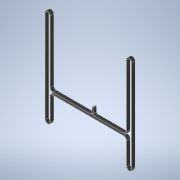
# Autodesk Inventor part: GT2 Belt
Saved by Autodesk Inventor 2022 (Build 260153000, 153)
## iProperties
Created: 2022-06-12
Part Number: GT2 Belt
Material: Generic
Document SubType Name: Modeling
Designer: Nick
Density: 1 g/cm^3
Appearance: Default
Author: Nick
Autodesk Inventor part; units mm, degrees
ref_plane "YZ Plane" through (0, 0, 0) normal (1, 0, 0) x (0, 1, 0)
ref_plane "XZ Plane" through (0, 0, 0) normal (0, 1, 0) x (-1, 0, 0)
ref_plane "XY Plane" through (0, 0, 0) normal (0, 0, 1) x (1, 0, 0)
ref_plane "Work Plane1" through (-134.646947, -237.429887, -822.943102) normal (0, 0, -1) x (0, -1, 0)
ref_plane "Work Plane3" through (-197.934852, -177.205039, -822.943102) normal (0, 1, 0) x (-1, 0, 0)
sketch "Sketch3" plane through (-197.934852, -177.205039, -822.943102) normal (0, 1, 0) x (-1, 0, 0)
  line L0 (0, 0) -> (1, 0)
  line L1 (1, 0) -> (1, -6)
  line L2 (1, -6) -> (0, -6)
  line L3 (0, -6) -> (0, 0)
  point P0 (-197.934852, 822.943102)
  dimension "d10" = 1
  dimension "d11" = 6
  constraints: 8 end point, 2 parallel, 1 horizontal, 1 perpendicular
  measures "d10" distance of L1.end L2.end
  measures "d11" distance of L0.end L1.end
sketch "Sketch1" plane through (-134.646947, -237.429887, -822.943102) normal (0, 0, -1) x (0, -1, 0)
  line L0 (0, 4.84) -> (-39.224848, 4.84)
  line L1 (-43.884848, 9.5) -> (-43.884848, 134.5)
  line L2 (-48.564848, 134.5) -> (-48.564848, 67.627904)
  line L3 (-48.564848, 61.127904) -> (-48.564848, 9.5)
  line L4 (-163, 4.84) -> (-53.224848, 4.84)
  line L5 (-163, -4.84) -> (0, -4.84)
  circle A0 centre (-53.224848, 9.5) radius 4.5 construction
  circle A1 centre (-39.224848, 9.5) radius 4.5 construction
  circle A2 centre (-53.224848, 134.5) radius 4.5
  circle A3 centre (-39.224848, 134.5) radius 4.5
  circle A4 centre (-163, 0) radius 4.5 construction
  circle A5 centre (-163, 144) radius 4.5
  arc A6 (1.927206, 148.234735) -> (2.866938, 147.664391) centre (2.386662, 147.93241) ccw construction
  arc A7 (3.109447, 147.709035) -> (2.866938, 147.664391) centre (3.006655, 147.586422) ccw construction
  arc A8 (3.424444, 147.420348) -> (3.109447, 147.709035) centre (0, 144) ccw construction
  arc A9 (3.401069, 147.174875) -> (3.424444, 147.420348) centre (3.31124, 147.307279) ccw construction
  arc A10 (3.401069, 147.174875) -> (4.051008, 146.288326) centre (3.709856, 146.719737) ccw construction
  arc A11 (4.292141, 146.236767) -> (4.051008, 146.288326) centre (4.150252, 146.162825) ccw construction
  arc A12 (4.472685, 145.849511) -> (4.292141, 146.236767) centre (0, 144) ccw construction
  arc A13 (4.35715, 145.631669) -> (4.472685, 145.849511) centre (4.324827, 145.788371) ccw construction
  arc A14 (4.35715, 145.631669) -> (4.618347, 144.563884) centre (4.468258, 145.093009) ccw construction
  arc A15 (4.821395, 144.423973) -> (4.618347, 144.563884) centre (4.66201, 144.409957) ccw construction
  arc A16 (4.839999, 143.997103) -> (4.821395, 144.423973) centre (0, 144) ccw construction
  arc A17 (4.649894, 143.840057) -> (4.839999, 143.997103) centre (4.679999, 143.997199) ccw construction
  arc A18 (4.649894, 143.840057) -> (4.482586, 142.753596) centre (4.546409, 143.29988) ccw construction
  arc A19 (4.616635, 142.546632) -> (4.482586, 142.753596) centre (4.464019, 142.594677) ccw construction
  arc A20 (4.470468, 142.145136) -> (4.616635, 142.546632) centre (0, 144) ccw construction
  arc A21 (4.234735, 142.072794) -> (4.470468, 142.145136) centre (4.322684, 142.206454) ccw construction
  arc A22 (4.234735, 142.072794) -> (3.664391, 141.133062) centre (3.93241, 141.613338) ccw construction
  arc A23 (3.709035, 140.890553) -> (3.664391, 141.133062) centre (3.586422, 140.993345) ccw construction
  arc A24 (3.420348, 140.575556) -> (3.709035, 140.890553) centre (0, 144) ccw construction
  arc A25 (3.174875, 140.598931) -> (3.420348, 140.575556) centre (3.307279, 140.68876) ccw construction
  arc A26 (3.174875, 140.598931) -> (2.288326, 139.948992) centre (2.719737, 140.290144) ccw construction
  arc A27 (2.236767, 139.707859) -> (2.288326, 139.948992) centre (2.162825, 139.849748) ccw construction
  arc A28 (1.849511, 139.527315) -> (2.236767, 139.707859) centre (0, 144) ccw construction
  arc A29 (1.631669, 139.64285) -> (1.849511, 139.527315) centre (1.788371, 139.675173) ccw construction
  arc A30 (1.631669, 139.64285) -> (0.563884, 139.381653) centre (1.093009, 139.531742) ccw construction
  arc A31 (0.423973, 139.178605) -> (0.563884, 139.381653) centre (0.409957, 139.33799) ccw construction
  arc A32 (-0.002897, 139.160001) -> (0.423973, 139.178605) centre (0, 144) ccw construction
  arc A33 (-0.159943, 139.350106) -> (-0.002897, 139.160001) centre (-0.002801, 139.320001) ccw construction
  arc A34 (-0.159943, 139.350106) -> (-1.246404, 139.517414) centre (-0.70012, 139.453591) ccw construction
  arc A35 (-1.453368, 139.383365) -> (-1.246404, 139.517414) centre (-1.405323, 139.535981) ccw construction
  arc A36 (-1.854864, 139.529532) -> (-1.453368, 139.383365) centre (0, 144) ccw construction
  arc A37 (-1.927206, 139.765265) -> (-1.854864, 139.529532) centre (-1.793546, 139.677316) ccw construction
  arc A38 (-1.927206, 139.765265) -> (-2.866938, 140.335609) centre (-2.386662, 140.06759) ccw construction
  arc A39 (-3.109447, 140.290965) -> (-2.866938, 140.335609) centre (-3.006655, 140.413578) ccw construction
  arc A40 (-3.424444, 140.579652) -> (-3.109447, 140.290965) centre (0, 144) ccw construction
  arc A41 (-3.401069, 140.825125) -> (-3.424444, 140.579652) centre (-3.31124, 140.692721) ccw construction
  arc A42 (-3.401069, 140.825125) -> (-4.051008, 141.711674) centre (-3.709856, 141.280263) ccw construction
  arc A43 (-4.292141, 141.763233) -> (-4.051008, 141.711674) centre (-4.150252, 141.837175) ccw construction
  arc A44 (-4.472685, 142.150489) -> (-4.292141, 141.763233) centre (0, 144) ccw construction
  arc A45 (-4.35715, 142.368331) -> (-4.472685, 142.150489) centre (-4.324827, 142.211629) ccw construction
  arc A46 (-4.35715, 142.368331) -> (-4.618347, 143.436116) centre (-4.468258, 142.906991) ccw construction
  arc A47 (-4.821395, 143.576027) -> (-4.618347, 143.436116) centre (-4.66201, 143.590043) ccw construction
  arc A48 (-4.839999, 144.002897) -> (-4.821395, 143.576027) centre (0, 144) ccw construction
  arc A49 (-4.649894, 144.159943) -> (-4.839999, 144.002897) centre (-4.679999, 144.002801) ccw construction
  arc A50 (-4.649894, 144.159943) -> (-4.482586, 145.246404) centre (-4.546409, 144.70012) ccw construction
  arc A51 (-4.616635, 145.453368) -> (-4.482586, 145.246404) centre (-4.464019, 145.405323) ccw construction
  arc A52 (-4.470468, 145.854864) -> (-4.616635, 145.453368) centre (0, 144) ccw construction
  arc A53 (-4.234735, 145.927206) -> (-4.470468, 145.854864) centre (-4.322684, 145.793546) ccw construction
  arc A54 (-4.234735, 145.927206) -> (-3.664391, 146.866938) centre (-3.93241, 146.386662) ccw construction
  arc A55 (-3.709035, 147.109447) -> (-3.664391, 146.866938) centre (-3.586422, 147.006655) ccw construction
  arc A56 (-3.420348, 147.424444) -> (-3.709035, 147.109447) centre (0, 144) ccw construction
  arc A57 (-3.174875, 147.401069) -> (-3.420348, 147.424444) centre (-3.307279, 147.31124) ccw construction
  arc A58 (-3.174875, 147.401069) -> (-2.288326, 148.051008) centre (-2.719737, 147.709856) ccw construction
  arc A59 (-2.236767, 148.292141) -> (-2.288326, 148.051008) centre (-2.162825, 148.150252) ccw construction
  arc A60 (-1.849511, 148.472685) -> (-2.236767, 148.292141) centre (0, 144) ccw construction
  arc A61 (-1.631669, 148.35715) -> (-1.849511, 148.472685) centre (-1.788371, 148.324827) ccw construction
  arc A62 (-1.631669, 148.35715) -> (-0.563884, 148.618347) centre (-1.093009, 148.468258) ccw construction
  arc A63 (-0.423973, 148.821395) -> (-0.563884, 148.618347) centre (-0.409957, 148.66201) ccw construction
  arc A64 (0.002897, 148.839999) -> (-0.423973, 148.821395) centre (0, 144) ccw construction
  arc A65 (0.159943, 148.649894) -> (0.002897, 148.839999) centre (0.002801, 148.679999) ccw construction
  arc A66 (0.159943, 148.649894) -> (1.246404, 148.482586) centre (0.70012, 148.546409) ccw construction
  arc A67 (1.453368, 148.616635) -> (1.246404, 148.482586) centre (1.405323, 148.464019) ccw construction
  arc A68 (1.854864, 148.470468) -> (1.453368, 148.616635) centre (0, 144) ccw construction
  arc A69 (1.927206, 148.234735) -> (1.854864, 148.470468) centre (1.793546, 148.322684) ccw construction
  arc A70 (3.655529, -2.878229) -> (2.878229, -3.655529) centre (3.252691, -3.252691) ccw construction
  arc A71 (2.863972, -3.9017) -> (2.878229, -3.655529) centre (2.769295, -3.772718) ccw construction
  arc A72 (2.508706, -4.139081) -> (2.863972, -3.9017) centre (0, 0) ccw construction
  arc A73 (2.275818, -4.058048) -> (2.508706, -4.139081) centre (2.425774, -4.002252) ccw construction
  arc A74 (2.275818, -4.058048) -> (1.260227, -4.478719) centre (1.760344, -4.249846) ccw construction
  arc A75 (1.152849, -4.700696) -> (1.260227, -4.478719) centre (1.114738, -4.545301) ccw construction
  arc A76 (0.733785, -4.784053) -> (1.152849, -4.700696) centre (0, 0) ccw construction
  arc A77 (0.549634, -4.620065) -> (0.733785, -4.784053) centre (0.709527, -4.625902) ccw construction
  arc A78 (0.549634, -4.620065) -> (-0.549634, -4.620065) centre (0, -4.6) ccw construction
  arc A79 (-0.733785, -4.784053) -> (-0.549634, -4.620065) centre (-0.709527, -4.625902) ccw construction
  arc A80 (-1.152849, -4.700696) -> (-0.733785, -4.784053) centre (0, 0) ccw construction
  arc A81 (-1.260227, -4.478719) -> (-1.152849, -4.700696) centre (-1.114738, -4.545301) ccw construction
  arc A82 (-1.260227, -4.478719) -> (-2.275818, -4.058048) centre (-1.760344, -4.249846) ccw construction
  arc A83 (-2.508706, -4.139081) -> (-2.275818, -4.058048) centre (-2.425774, -4.002252) ccw construction
  arc A84 (-2.863972, -3.9017) -> (-2.508706, -4.139081) centre (0, 0) ccw construction
  arc A85 (-2.878229, -3.655529) -> (-2.863972, -3.9017) centre (-2.769295, -3.772718) ccw construction
  arc A86 (-2.878229, -3.655529) -> (-3.655529, -2.878229) centre (-3.252691, -3.252691) ccw construction
  arc A87 (-3.9017, -2.863972) -> (-3.655529, -2.878229) centre (-3.772718, -2.769295) ccw construction
  arc A88 (-4.139081, -2.508706) -> (-3.9017, -2.863972) centre (0, 0) ccw construction
  arc A89 (-4.058048, -2.275818) -> (-4.139081, -2.508706) centre (-4.002252, -2.425774) ccw construction
  arc A90 (-4.058048, -2.275818) -> (-4.478719, -1.260227) centre (-4.249846, -1.760344) ccw construction
  arc A91 (-4.700696, -1.152849) -> (-4.478719, -1.260227) centre (-4.545301, -1.114738) ccw construction
  arc A92 (-4.784053, -0.733785) -> (-4.700696, -1.152849) centre (0, 0) ccw construction
  arc A93 (-4.620065, -0.549634) -> (-4.784053, -0.733785) centre (-4.625902, -0.709527) ccw construction
  arc A94 (-4.620065, -0.549634) -> (-4.620065, 0.549634) centre (-4.6, 0) ccw construction
  arc A95 (-4.784053, 0.733785) -> (-4.620065, 0.549634) centre (-4.625902, 0.709527) ccw construction
  arc A96 (-4.700696, 1.152849) -> (-4.784053, 0.733785) centre (0, 0) ccw construction
  arc A97 (-4.478719, 1.260227) -> (-4.700696, 1.152849) centre (-4.545301, 1.114738) ccw construction
  arc A98 (-4.478719, 1.260227) -> (-4.058048, 2.275818) centre (-4.249846, 1.760344) ccw construction
  arc A99 (-4.139081, 2.508706) -> (-4.058048, 2.275818) centre (-4.002252, 2.425774) ccw construction
  arc A100 (-3.9017, 2.863972) -> (-4.139081, 2.508706) centre (0, 0) ccw construction
  arc A101 (-3.655529, 2.878229) -> (-3.9017, 2.863972) centre (-3.772718, 2.769295) ccw construction
  arc A102 (-3.655529, 2.878229) -> (-2.878229, 3.655529) centre (-3.252691, 3.252691) ccw construction
  arc A103 (-2.863972, 3.9017) -> (-2.878229, 3.655529) centre (-2.769295, 3.772718) ccw construction
  arc A104 (-2.508706, 4.139081) -> (-2.863972, 3.9017) centre (0, 0) ccw construction
  arc A105 (-2.275818, 4.058048) -> (-2.508706, 4.139081) centre (-2.425774, 4.002252) ccw construction
  arc A106 (-2.275818, 4.058048) -> (-1.260227, 4.478719) centre (-1.760344, 4.249846) ccw construction
  arc A107 (-1.152849, 4.700696) -> (-1.260227, 4.478719) centre (-1.114738, 4.545301) ccw construction
  arc A108 (-0.733785, 4.784053) -> (-1.152849, 4.700696) centre (0, 0) ccw construction
  arc A109 (-0.549634, 4.620065) -> (-0.733785, 4.784053) centre (-0.709527, 4.625902) ccw construction
  arc A110 (-0.549634, 4.620065) -> (0.549634, 4.620065) centre (0, 4.6) ccw construction
  arc A111 (0.733785, 4.784053) -> (0.549634, 4.620065) centre (0.709527, 4.625902) ccw construction
  arc A112 (1.152849, 4.700696) -> (0.733785, 4.784053) centre (0, 0) ccw construction
  arc A113 (1.260227, 4.478719) -> (1.152849, 4.700696) centre (1.114738, 4.545301) ccw construction
  arc A114 (1.260227, 4.478719) -> (2.275818, 4.058048) centre (1.760344, 4.249846) ccw construction
  arc A115 (2.508706, 4.139081) -> (2.275818, 4.058048) centre (2.425774, 4.002252) ccw construction
  arc A116 (2.863972, 3.9017) -> (2.508706, 4.139081) centre (0, 0) ccw construction
  arc A117 (2.878229, 3.655529) -> (2.863972, 3.9017) centre (2.769295, 3.772718) ccw construction
  arc A118 (2.878229, 3.655529) -> (3.655529, 2.878229) centre (3.252691, 3.252691) ccw construction
  arc A119 (3.9017, 2.863972) -> (3.655529, 2.878229) centre (3.772718, 2.769295) ccw construction
  arc A120 (4.139081, 2.508706) -> (3.9017, 2.863972) centre (0, 0) ccw construction
  arc A121 (4.058048, 2.275818) -> (4.139081, 2.508706) centre (4.002252, 2.425774) ccw construction
  arc A122 (4.058048, 2.275818) -> (4.478719, 1.260227) centre (4.249846, 1.760344) ccw construction
  arc A123 (4.700696, 1.152849) -> (4.478719, 1.260227) centre (4.545301, 1.114738) ccw construction
  arc A124 (4.784053, 0.733785) -> (4.700696, 1.152849) centre (0, 0) ccw construction
  arc A125 (4.620065, 0.549634) -> (4.784053, 0.733785) centre (4.625902, 0.709527) ccw construction
  arc A126 (4.620065, 0.549634) -> (4.620065, -0.549634) centre (4.6, 0) ccw construction
  arc A127 (4.784053, -0.733785) -> (4.620065, -0.549634) centre (4.625902, -0.709527) ccw construction
  arc A128 (4.700696, -1.152849) -> (4.784053, -0.733785) centre (0, 0) ccw construction
  arc A129 (4.478719, -1.260227) -> (4.700696, -1.152849) centre (4.545301, -1.114738) ccw construction
  arc A130 (4.478719, -1.260227) -> (4.058048, -2.275818) centre (4.249846, -1.760344) ccw construction
  arc A131 (4.139081, -2.508706) -> (4.058048, -2.275818) centre (4.002252, -2.425774) ccw construction
  arc A132 (3.9017, -2.863972) -> (4.139081, -2.508706) centre (0, 0) ccw construction
  arc A133 (3.655529, -2.878229) -> (3.9017, -2.863972) centre (3.772718, -2.769295) ccw construction
  arc A134 (-39.224848, 139.16) -> (-43.884848, 134.5) centre (-39.224848, 134.5) ccw
  arc A135 (-48.564848, 134.5) -> (-53.224848, 139.16) centre (-53.224848, 134.5) ccw
  arc A136 (-163, 148.84) -> (-163, 139.16) centre (-163, 144) ccw
  line L6 (-163, 139.16) -> (-53.224848, 139.16)
  arc A137 (-43.884848, 9.5) -> (-39.224848, 4.84) centre (-39.224848, 9.5) ccw
  arc A138 (-53.224848, 4.84) -> (-48.564848, 9.5) centre (-53.224848, 9.5) ccw
  arc A139 (-163, 4.84) -> (-163, -4.84) centre (-163, 0) ccw
  line L7 (-48.724848, 70.377904) -> (-42.724848, 70.377904) construction
  line L8 (-48.724848, 67.627904) -> (-48.724848, 70.377904) construction
  arc A140 (-50.724848, 65.627904) -> (-48.724848, 67.627904) centre (-50.724848, 67.627904) ccw construction
  line L9 (-60.224848, 65.627904) -> (-50.724848, 65.627904) construction
  line L10 (-60.224848, 63.127904) -> (-60.224848, 65.627904) construction
  line L11 (-50.724848, 63.127904) -> (-60.224848, 63.127904) construction
  arc A141 (-48.724848, 61.127904) -> (-50.724848, 63.127904) centre (-50.724848, 61.127904) ccw construction
  line L12 (-48.724848, 58.377904) -> (-48.724848, 61.127904) construction
  line L13 (-42.724848, 58.377904) -> (-48.724848, 58.377904) construction
  line L14 (-42.724848, 70.377904) -> (-42.724848, 58.377904) construction
  arc A142 (-48.564848, 61.127904) -> (-50.724848, 63.287904) centre (-50.724848, 61.127904) ccw
  arc A143 (-50.724848, 65.467904) -> (-48.564848, 67.627904) centre (-50.724848, 67.627904) ccw
  line L15 (-50.724848, 63.287904) -> (-60.224848, 63.287904)
  line L16 (-50.724848, 65.467904) -> (-60.224848, 65.467904)
  line L17 (-39.224848, 139.16) -> (0, 139.16)
  line L18 (0, 148.84) -> (-163, 148.84)
  arc A144 (0, 139.16) -> (0, 148.84) centre (0, 144) ccw
  arc A145 (0, -4.84) -> (0, 4.84) centre (0, 0) ccw
  point P0 (-237.429887, -134.646947)
sweep "Sweep3" add profiles "Sketch3" path "Sketch1" path curves L15 A142 L3 A138 L4 A139 L5 A145 L0 A137 L1 A134 L17 A144 L18 A136 L6 A135 L2 A143 L16
body "Solid4"
